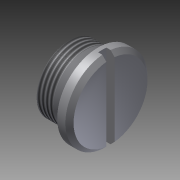
# Autodesk Inventor part: 13_1087_042
Saved by Autodesk Inventor 2014 SP1 (Build 180222100, 222)
## iProperties
Created: 2013-10-21
Part Number: 13_1087_042
Material: Allgemein
Document SubType Name: Modeling
Designer: vogel
Density: 1 g/cm^3
Appearance: Vorgabe
Author: vogel
Autodesk Inventor part; units mm, degrees
ref_plane "YZ Plane" through (0, 0, 0) normal (1, 0, 0) x (0, 1, 0)
ref_plane "XZ Plane" through (0, 0, 0) normal (0, 1, 0) x (-1, 0, 0)
ref_plane "XY Plane" through (0, 0, 0) normal (0, 0, 1) x (1, 0, 0)
sketch "Skizze1" plane through (0, 0, 0) normal (0, 0, 1) x (1, 0, 0)
  line L0 (-6, 0) -> (1, 0) projected
  line L1 (0, -1) -> (0, 6) projected
  line L2 (0, 0) -> (0, 5)
  line L3 (0, 5) -> (-1.5, 5)
  line L4 (-1.5, 5) -> (-1.5, 3.5)
  line L5 (-1.5, 3.5) -> (-2.5, 3.5)
  line L6 (-2.5, 3.5) -> (-3, 4)
  line L7 (-3, 4) -> (-5, 4)
  line L8 (-5, 4) -> (-5, 0)
  line L9 (-5, 0) -> (0, 0)
  dimension "d0" = 8
  dimension "d1" = 10
  dimension "d2" = 1.5
  dimension "d3" = 1
  dimension "d4" = 7
  dimension "d5" = 45
  dimension "d6" = 5
  constraints: 16 end point, 3 parallel, 2 perpendicular, 2 point on line, 1 collinear
  measures "d0" diameter of L7 L0
  measures "d1" diameter of L3 L0
  measures "d2" distance of L2.end L3.end
  measures "d3" distance of L4.end L5.end
  measures "d4" diameter of L5 L0
  measures "d5" angle of L5 L6
  measures "d6" distance between parallel lines of L8 L1
revolve "Umdrehung1" add sketch "Skizze1" angle 360 about axis through (-10, 0, 0) along (1, 0, 0)
sketch "Skizze2" plane through (0, 0, 0) normal (1, 0, 0) x (0, 0, -1)
  line L0 (-7.1847, 0.5) -> (7.4374, 0.5)
  line L1 (7.4374, 0.5) -> (7.4374, -0.5)
  line L2 (7.4374, -0.5) -> (-7.1847, -0.5)
  line L3 (-7.1847, -0.5) -> (-7.1847, 0.5)
  line L4 (0, -7) -> (0, 7) projected
  line L5 (10.3619, 0) -> (-10.1091, 0) projected
  dimension "d8" = 1
  constraints: 8 end point, 2 parallel, 1 horizontal, 1 perpendicular, 1 other
  measures "d8" distance between parallel lines of L2 L0
extrude "Extrusion1" cut sketch "Skizze2" against normal blind 1
thread "Gewinde1" size "M8x0.5" class "6g" standard "ANSI Metric M Profile" full length
chamfer "Fase1" distance 0.5 angle 45 3 edges at (0, -5, 0) (0, 3.7081, -3.3541) (0, 3.7081, 3.3541)
